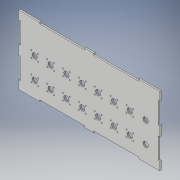
# Autodesk Inventor part: case_back
Saved by Autodesk Inventor 2019 (Build 230136000, 136)
## iProperties
Created: 2019-07-12
Part Number: case_back
Material: Generic
Document SubType Name: Modeling
Designer: Lino P
Density: 1 g/cm^3
Appearance: Default
Author: Lino P
Autodesk Inventor part; units mm, degrees
ref_plane "YZ Plane" through (0, 0, 0) normal (1, 0, 0) x (0, 1, 0)
ref_plane "XZ Plane" through (0, 0, 0) normal (0, 1, 0) x (-1, 0, 0)
ref_plane "XY Plane" through (0, 0, 0) normal (0, 0, 1) x (1, 0, 0)
sketch "Sketch1" plane through (0, 0, 0) normal (0, 0, 1) x (1, 0, 0)
  line L0 (-15, 84.2) -> (252, 84.2)
  line L1 (252, 84.2) -> (252, -46)
  line L2 (252, -46) -> (-15, -46)
  line L3 (-15, -46) -> (-15, 84.2)
  line L4 (118.5, 84.2) -> (118.5, -46) construction
  line L5 (25, 84.2) -> (110, 84.2)
  line L6 (110, 84.2) -> (110, 81.2)
  line L7 (110, 81.2) -> (25, 81.2)
  line L8 (25, 81.2) -> (25, 84.2)
  line L9 (212, 84.2) -> (127, 84.2)
  line L10 (127, 84.2) -> (127, 81.2)
  line L11 (127, 81.2) -> (212, 81.2)
  line L12 (212, 81.2) -> (212, 84.2)
  line L13 (25, -46) -> (110, -46)
  line L14 (110, -46) -> (110, -43)
  line L15 (110, -43) -> (25, -43)
  line L16 (25, -43) -> (25, -46)
  line L17 (212, -43) -> (212, -46)
  line L18 (127, -46) -> (127, -43)
  line L19 (127, -43) -> (212, -43)
  line L20 (212, -46) -> (127, -46)
  line L21 (-15, 24.2) -> (252, 24.2) construction
  circle A0 centre (15.4749, 24.2) radius 5
  line L22 (6.5749, 15.3) -> (24.3749, 15.3) construction
  line L23 (24.3749, 15.3) -> (24.3749, 33.1) construction
  line L24 (24.3749, 33.1) -> (6.5749, 33.1) construction
  line L25 (6.5749, 33.1) -> (6.5749, 15.3) construction
  circle A1 centre (9.1249, 30.55) radius 1.05
  line L26 (9.1249, 30.55) -> (9.1249, 31.6) construction
  line L27 (9.1249, 30.55) -> (8.0749, 30.55) construction
  line L28 (15.4749, 33.1) -> (15.4749, 15.3) construction
  line L29 (6.5749, 24.2) -> (24.3749, 24.2) construction
  circle A2 centre (21.8249, 30.55) radius 1.05
  line L30 (21.8249, 30.55) -> (21.8249, 31.6) construction
  line L31 (21.8249, 30.55) -> (22.8749, 30.55) construction
  circle A3 centre (9.1249, 17.85) radius 1.05
  line L32 (9.1249, 17.85) -> (9.1249, 16.8) construction
  line L33 (9.1249, 17.85) -> (8.0749, 17.85) construction
  line L34 (21.8249, 17.85) -> (21.8249, 16.8) construction
  line L35 (21.8249, 17.85) -> (22.8749, 17.85) construction
  circle A4 centre (21.8249, 17.85) radius 1.05
  circle A5 centre (45.4749, 24.2) radius 5
  circle A6 centre (75.4749, 24.2) radius 5
  circle A7 centre (105.4749, 24.2) radius 5
  circle A8 centre (135.4749, 24.2) radius 5
  circle A9 centre (165.4749, 24.2) radius 5
  circle A10 centre (195.4749, 24.2) radius 5
  circle A11 centre (225.4749, 24.2) radius 5
  circle A12 centre (15.4749, -15.8) radius 5
  circle A13 centre (45.4749, -15.8) radius 5
  circle A14 centre (75.4749, -15.8) radius 5
  circle A15 centre (105.4749, -15.8) radius 5
  circle A16 centre (135.4749, -15.8) radius 5
  circle A17 centre (165.4749, -15.8) radius 5
  circle A18 centre (195.4749, -15.8) radius 5
  circle A19 centre (225.4749, -15.8) radius 5
  circle A20 centre (9.1249, -9.45) radius 1.05
  circle A21 centre (21.8249, -9.45) radius 1.05
  circle A22 centre (21.8249, -22.15) radius 1.05
  circle A23 centre (9.1249, -22.15) radius 1.05
  circle A24 centre (39.1249, 30.55) radius 1.05
  circle A25 centre (51.8249, 30.55) radius 1.05
  circle A26 centre (51.8249, 17.85) radius 1.05
  circle A27 centre (39.1249, 17.85) radius 1.05
  circle A28 centre (39.1249, -9.45) radius 1.05
  circle A29 centre (51.8249, -9.45) radius 1.05
  circle A30 centre (51.8249, -22.15) radius 1.05
  circle A31 centre (39.1249, -22.15) radius 1.05
  circle A32 centre (69.1249, 30.55) radius 1.05
  circle A33 centre (81.8249, 30.55) radius 1.05
  circle A34 centre (81.8249, 17.85) radius 1.05
  circle A35 centre (69.1249, 17.85) radius 1.05
  circle A36 centre (69.1249, -9.45) radius 1.05
  circle A37 centre (81.8249, -9.45) radius 1.05
  circle A38 centre (81.8249, -22.15) radius 1.05
  circle A39 centre (69.1249, -22.15) radius 1.05
  circle A40 centre (99.1249, 30.55) radius 1.05
  circle A41 centre (111.8249, 30.55) radius 1.05
  circle A42 centre (111.8249, 17.85) radius 1.05
  circle A43 centre (99.1249, 17.85) radius 1.05
  circle A44 centre (99.1249, -9.45) radius 1.05
  circle A45 centre (111.8249, -9.45) radius 1.05
  circle A46 centre (111.8249, -22.15) radius 1.05
  circle A47 centre (99.1249, -22.15) radius 1.05
  circle A48 centre (129.1249, 30.55) radius 1.05
  circle A49 centre (141.8249, 30.55) radius 1.05
  circle A50 centre (141.8249, 17.85) radius 1.05
  circle A51 centre (129.1249, 17.85) radius 1.05
  circle A52 centre (129.1249, -9.45) radius 1.05
  circle A53 centre (141.8249, -9.45) radius 1.05
  circle A54 centre (141.8249, -22.15) radius 1.05
  circle A55 centre (129.1249, -22.15) radius 1.05
  circle A56 centre (159.1249, 30.55) radius 1.05
  circle A57 centre (171.8249, 30.55) radius 1.05
  circle A58 centre (171.8249, 17.85) radius 1.05
  circle A59 centre (159.1249, 17.85) radius 1.05
  circle A60 centre (159.1249, -9.45) radius 1.05
  circle A61 centre (171.8249, -9.45) radius 1.05
  circle A62 centre (171.8249, -22.15) radius 1.05
  circle A63 centre (159.1249, -22.15) radius 1.05
  circle A64 centre (189.1249, 30.55) radius 1.05
  circle A65 centre (201.8249, 30.55) radius 1.05
  circle A66 centre (201.8249, 17.85) radius 1.05
  circle A67 centre (189.1249, 17.85) radius 1.05
  circle A68 centre (189.1249, -9.45) radius 1.05
  circle A69 centre (201.8249, -9.45) radius 1.05
  circle A70 centre (201.8249, -22.15) radius 1.05
  circle A71 centre (189.1249, -22.15) radius 1.05
  line L36 (252, 68.2) -> (249, 68.2)
  line L37 (249, 68.2) -> (249, 28.2)
  line L38 (249, 28.2) -> (252, 28.2)
  line L39 (252, 28.2) -> (252, 68.2)
  line L40 (-15, 19.1) -> (252, 19.1) construction
  line L41 (252, -30) -> (249, -30)
  line L42 (249, -30) -> (249, 10)
  line L43 (249, 10) -> (252, 10)
  line L44 (252, 10) -> (252, -30)
  line L45 (-15, 68.2) -> (-12, 68.2)
  line L46 (-12, 68.2) -> (-12, 28.2)
  line L47 (-12, 28.2) -> (-15, 28.2)
  line L48 (-15, 28.2) -> (-15, 68.2)
  line L49 (-15, -30) -> (-12, -30)
  line L50 (-12, -30) -> (-12, 10)
  line L51 (-15, 10) -> (-15, -30)
  line L52 (-12, 10) -> (-15, 10)
  point P0 (0, 0)
  point P1 (-15, 77.349)
  point P2 (9.1249, -8.4)
  point P3 (8.0749, -9.45)
  point P4 (21.8249, -8.4)
  point P5 (22.8749, -9.45)
  point P6 (21.8249, -23.2)
  point P7 (22.8749, -22.15)
  point P8 (9.1249, -23.2)
  point P9 (8.0749, -22.15)
  point P10 (39.1249, 31.6)
  point P11 (38.0749, 30.55)
  point P12 (51.8249, 31.6)
  point P13 (52.8749, 30.55)
  point P14 (51.8249, 16.8)
  point P15 (52.8749, 17.85)
  point P16 (39.1249, 16.8)
  point P17 (38.0749, 17.85)
  point P18 (39.1249, -8.4)
  point P19 (38.0749, -9.45)
  point P20 (51.8249, -8.4)
  point P21 (52.8749, -9.45)
  point P22 (51.8249, -23.2)
  point P23 (52.8749, -22.15)
  point P24 (39.1249, -23.2)
  point P25 (38.0749, -22.15)
  point P26 (69.1249, 31.6)
  point P27 (68.0749, 30.55)
  point P28 (81.8249, 31.6)
  point P29 (82.8749, 30.55)
  point P30 (81.8249, 16.8)
  point P31 (82.8749, 17.85)
  point P32 (69.1249, 16.8)
  point P33 (68.0749, 17.85)
  point P34 (69.1249, -8.4)
  point P35 (68.0749, -9.45)
  point P36 (81.8249, -8.4)
  point P37 (82.8749, -9.45)
  point P38 (81.8249, -23.2)
  point P39 (82.8749, -22.15)
  point P40 (69.1249, -23.2)
  point P41 (68.0749, -22.15)
  point P42 (99.1249, 31.6)
  point P43 (98.0749, 30.55)
  point P44 (111.8249, 31.6)
  point P45 (112.8749, 30.55)
  point P46 (111.8249, 16.8)
  point P47 (112.8749, 17.85)
  point P48 (99.1249, 16.8)
  point P49 (98.0749, 17.85)
  point P50 (99.1249, -8.4)
  point P51 (98.0749, -9.45)
  point P52 (111.8249, -8.4)
  point P53 (112.8749, -9.45)
  point P54 (111.8249, -23.2)
  point P55 (112.8749, -22.15)
  point P56 (99.1249, -23.2)
  point P57 (98.0749, -22.15)
  point P58 (129.1249, 31.6)
  point P59 (128.0749, 30.55)
  point P60 (141.8249, 31.6)
  point P61 (142.8749, 30.55)
  point P62 (141.8249, 16.8)
  point P63 (142.8749, 17.85)
  point P64 (129.1249, 16.8)
  point P65 (128.0749, 17.85)
  point P66 (129.1249, -8.4)
  point P67 (128.0749, -9.45)
  point P68 (141.8249, -8.4)
  point P69 (142.8749, -9.45)
  point P70 (141.8249, -23.2)
  point P71 (142.8749, -22.15)
  point P72 (129.1249, -23.2)
  point P73 (128.0749, -22.15)
  point P74 (159.1249, 31.6)
  point P75 (158.0749, 30.55)
  point P76 (171.8249, 31.6)
  point P77 (172.8749, 30.55)
  point P78 (171.8249, 16.8)
  point P79 (172.8749, 17.85)
  point P80 (159.1249, 16.8)
  point P81 (158.0749, 17.85)
  point P82 (159.1249, -8.4)
  point P83 (158.0749, -9.45)
  point P84 (171.8249, -8.4)
  point P85 (172.8749, -9.45)
  point P86 (171.8249, -23.2)
  point P87 (172.8749, -22.15)
  point P88 (159.1249, -23.2)
  point P89 (158.0749, -22.15)
  point P90 (189.1249, 31.6)
  point P91 (188.0749, 30.55)
  point P92 (201.8249, 31.6)
  point P93 (202.8749, 30.55)
  point P94 (201.8249, 16.8)
  point P95 (202.8749, 17.85)
  point P96 (189.1249, 16.8)
  point P97 (188.0749, 17.85)
  point P98 (189.1249, -8.4)
  point P99 (188.0749, -9.45)
  point P100 (201.8249, -8.4)
  point P101 (202.8749, -9.45)
  point P102 (201.8249, -23.2)
  point P103 (202.8749, -22.15)
  point P104 (189.1249, -23.2)
  point P105 (188.0749, -22.15)
  point P106 (11.5251, 24.2)
  point P107 (11.5251, -15.8)
  dimension "d41" = 3
  dimension "d42" = 40
  dimension "d43" = 85
  dimension "d46" = 10
  dimension "d47" = 17.8
  dimension "d48" = 17.8
  dimension "d50" = 1.5
  dimension "d51" = 2.1
  dimension "d52" = 1.5
  dimension "d55" = 30
  dimension "d58" = 40
  dimension "d63" = 40
  dimension "d66" = 30
  dimension "d71" = 267
  dimension "d72" = 130.2
  dimension "d73" = 60
  dimension "d74" = 124.2
  dimension "d76" = 124.2
  dimension "d77" = 3
  dimension "d78" = 40
  dimension "d79" = 16
  constraints: 112 point on circle, 106 end point, 72 centre point, 21 symmetric about line, 9 midpoint, 8 parallel, 6 horizontal, 5 perpendicular, 4 point on line, 3 vertical, 239 other
  measures "d41" distance of L5.end L6.end
  measures "d42" distance between parallel lines of L8 L3
  measures "d43" distance between parallel lines of L8 L6
  measures "d46" diameter of A0
  measures "d47" distance of L24.end L23.end
  measures "d48" distance of L23.end L22.end
  measures "d50" distance from line of L25 L27.end
  measures "d51" diameter of A1
  measures "d52" distance from line of L24 L26.end
  measures "d55" distance of A0.centre A5.centre
  measures "d58" distance of A0.centre A12.centre
  measures "d63" distance of L26.start A20.centre
  measures "d66" distance of L26.start A24.centre
  measures "d71" distance between parallel lines of L1 L3
  measures "d72" distance between parallel lines of L0 L2
  measures "d73" distance between parallel lines of L0 L21
  measures "d74" distance between parallel lines of L7 L15
  measures "d76" distance between parallel lines of L11 L19
  measures "d77" distance of L38.end L37.end
  measures "d78" distance of L37.end L36.end
  measures "d79" distance from line of L0 L36.end
extrude "Extrusion3" add sketch "Sketch1" along normal blind 3 contours L0 L8 L7 L6 L10 L11 L12 L1 L36 L37 L38 L43 L42 L41 L2 L17 L19 L18 L14 L15 L16 L3 L49 L50 L52 L47 L46 L45
body "Solid2"
